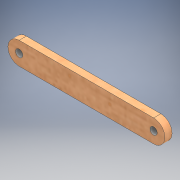
# Autodesk Inventor part: portabateria
Saved by Autodesk Inventor 2018 (Build 220112000, 112)
## iProperties
Created: 2017-05-11
Part Number: portabateria
Material: Generic
Document SubType Name: Modeling
Designer: Vidal Villegas
Density: 1 g/cm^3
Appearance: Default
Author: Vidal Villegas
Autodesk Inventor part; units mm, degrees
ref_plane "YZ Plane" through (0, 0, 0) normal (1, 0, 0) x (0, 1, 0)
ref_plane "XZ Plane" through (0, 0, 0) normal (0, 1, 0) x (-1, 0, 0)
ref_plane "XY Plane" through (0, 0, 0) normal (0, 0, 1) x (1, 0, 0)
sketch "Sketch1" plane through (0, 0, 0) normal (0, 1, 0) x (-1, 0, 0)
  circle A0 centre (55.9159, 0.1374) radius 1.6
  circle A1 centre (-3.8401, 0.1374) radius 1.6
  line L0 (55.9159, 5.1374) -> (-3.8401, 5.1374)
  line L1 (-3.8401, -4.8626) -> (55.9159, -4.8626)
  arc A2 (55.9159, -4.8626) -> (55.9159, 5.1374) centre (55.9159, 0.1374) ccw
  arc A3 (-3.8401, 5.1374) -> (-3.8401, -4.8626) centre (-3.8401, 0.1374) ccw
  point P0 (0, 0)
  dimension "d0" = 3.2
  dimension "d1" = 3.2
  dimension "d2" = 59.756
  dimension "d3" = 5
  dimension "d4" = 5
  constraints: 4 centre point, 4 end point, 4 point on circle, 2 equal radius, 1 horizontal, 1 parallel, 1 tangent
  measures "d0" diameter of A0
  measures "d1" diameter of A1
  measures "d2" distance of A1.centre A0.centre
  measures "d3" distance of L1.start A1.centre
  measures "d4" distance of L0.end A1.centre
extrude "Extrusion1" add sketch "Sketch1" along normal blind 3.2
equation "\"d4\" = d3"
body "Solid1"
